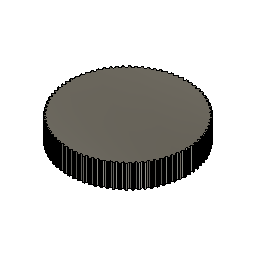
gear_82z (Autodesk Fusion 360 design; units mm, degrees)
Autodesk Fusion 360 part; units mm, degrees
sketch "Sketch1" plane through (0, 0, 0) normal (0, 0, 1) x (1, 0, 0) in component "gt2 pulley"
  circle A0 centre (0, 0) radius 26.1014 construction
  circle A1 centre (0, 0) radius 25.0974 construction
  line L0 (0, 0) -> (0, 26.1014) construction
  line L1 (0, 0) -> (0.9998, 26.0823) construction
  line L2 (0, 0) -> (1.4048, 26.0636) construction
  circle A2 centre (0, 0) radius 25.8474 construction
  arc A3 (0.396, 25.7111) -> (0.473, 25.4136) centre (1.3911, 25.8099) ccw
  circle A4 centre (0, 0) radius 25.6974 construction
  arc A5 (0.2481, 25.8462) -> (0, 25.8474) centre (0, 0) ccw
  arc A6 (0.396, 25.7111) -> (0.2481, 25.8462) centre (0.2468, 25.6962) ccw
  arc A7 (0.473, 25.4136) -> (0.9613, 25.079) centre (0.9826, 25.6336) ccw
  arc A8 (0, 25.8474) -> (-0.2481, 25.8462) centre (0, 0) ccw
  arc A9 (-0.2481, 25.8462) -> (-0.396, 25.7111) centre (-0.2468, 25.6962) ccw
  arc A10 (-0.473, 25.4136) -> (-0.396, 25.7111) centre (-1.3911, 25.8099) ccw
  arc A11 (-0.9613, 25.079) -> (-0.473, 25.4136) centre (-0.9826, 25.6336) ccw
  arc A12 (0.9613, 25.079) -> (-0.9613, 25.079) centre (0, 0) ccw
  point P0 (1.3911, 25.8099)
  point P1 (0, 25.8474)
  dimension "d18" = 52.2028
  dimension "d19" = 2.195
  dimension "d22" = 1.004
  dimension "d24" = 0.75
  dimension "d26" = 1
  dimension "d27" = 0.15
  dimension "d28" = 0.15
  dimension "d47" = 0.555
  dimension "d52" = 3.812
  constraint coincident A0.centre A1.centre
  constraint coincident A0 L0.end
  constraint vertical L0
  constraint coincident A0 L1.end
  constraint coincident A0 L2.end
  constraint concentric A1 A2
  constraint coincident A1 A7.end
  constraint coincident L1 A7.end
  constraint coincident A2 P0
  constraint coincident L2 P0
  constraint coincident P0 A3.centre
  constraint coincident A2 P1
  constraint coincident L0 P1
  constraint concentric A2 A4
  constraint coincident P1 A5.end
  constraint coincident A4 A6.centre
  constraint coincident A3.start A6.start
  constraint tangent A3 A6
  constraint tangent A3 A7
  constraint symmetric L0 A7.end A11.start
  constraint symmetric L0 A3.start A9.end
  constraint symmetric L0 A3.end A10.start
  constraint symmetric L0 A3 A10
  constraint symmetric L0 A5.start A8.end
  constraint symmetric L0 P1 A5.end
  constraint symmetric L0 A5 A8
  constraint symmetric L0 A6 A9
  constraint symmetric L0 A7 A11
  constraint coincident A1 A11.start
  constraint tangent A1 A7
  constraint coincident L1 A7.centre
  measures "d18" diameter of A0
  measures "d19" angle of L0 L1
  measures "d22" distance of A0 A1
  measures "d24" distance of A1 A2
  measures "d26" radius of A3
  measures "d27" distance of A2 A4
  measures "d28" radius of A6
  measures "d47" radius of A7
extrude "Extrude1" add sketch "Sketch1" along normal blind 10 makes body 1
pattern_circular "C-Pattern1" count 82 over 360 about axis through (0, 0, 1.75) along (0, 0, 1) of bodies 1 makes body 2 at (-2.0277, 25.0154, 6.6667) makes body 3 at (-3.9367, 24.7867, 6.6667) makes body 4 at (-5.8225, 24.4127, 6.6667) makes body 5 at (-8.2819, 23.6915, 6.6667) makes body 6 at (-8.6841, 23.5471, 3.3333) makes body 7 at (-11.6124, 22.2493, 6.6667) makes body 8 at (-12.1768, 21.9455, 3.3333) makes body 9 at (-13.821, 20.949, 6.6667) makes body 10 at (-16.0503, 19.2942, 6.6667) makes body 11 at (-16.8569, 18.5937, 3.3333) makes body 12 at (-18.8075, 16.618, 6.6667) makes body 13 at (-20.2791, 14.7864, 6.6667) makes body 14 at (-21.1238, 13.5523, 6.6667) makes body 15 at (-21.6814, 12.6411, 3.3333) makes body 16 at (-22.5854, 10.9443, 6.6667) makes body 17 at (-23.3569, 9.1833, 3.3333) makes body 18 at (-24.3877, 5.9264, 6.6667) makes body 19 at (-24.7698, 4.0421, 6.6667) makes body 20 at (-25.0065, 2.1342, 6.6667) makes body 21 at (-25.0965, 0.2137, 6.6667) makes body 22 at (-25.0965, -0.2137, 3.3333) makes body 23 at (-25.0065, -2.1342, 3.3333) makes body 24 at (-24.485, -5.5103, 6.6667) makes body 25 at (-23.9914, -7.3684, 6.6667) makes body 26 at (-23.4343, -8.9841, 6.6667) makes body 27 at (-22.5854, -10.9443, 6.6667) makes body 28 at (-21.6814, -12.6411, 6.6667) makes body 29 at (-21.463, -13.0084, 3.3333) makes body 30 at (-19.6315, -15.636, 6.6667) makes body 31 at (-18.2307, -17.2488, 6.6667) makes body 32 at (-17.9344, -17.5567, 3.3333) makes body 33 at (-16.5378, -18.878, 6.6667) makes body 34 at (-14.8726, -20.216, 6.6667) makes body 35 at (-12.3632, -21.841, 6.6667) makes body 36 at (-10.655, -22.7234, 6.6667) makes body 37 at (-8.6841, -23.5471, 6.6667) makes body 38 at (-6.8561, -24.1428, 6.6667) makes body 39 at (-6.4441, -24.256, 3.3333) makes body 40 at (-4.5684, -24.6781, 3.3333) makes body 41 at (-1.1748, -25.0699, 6.6667) makes body 42 at (-0.1068, -25.0972, 6.6667) makes body 43 at (1.1748, -25.0699, 3.3333) makes body 44 at (3.9367, -24.7867, 6.6667) makes body 45 at (5.8225, -24.4127, 6.6667) makes body 46 at (8.2819, -23.6915, 6.6667) makes body 47 at (8.6841, -23.5471, 3.3333) makes body 48 at (11.6124, -22.2493, 6.6667) makes body 49 at (12.917, -21.5182, 6.6667) makes body 50 at (13.821, -20.949, 6.6667) makes body 51 at (16.0503, -19.2942, 6.6667) makes body 52 at (16.8569, -18.5937, 3.3333) makes body 53 at (19.2257, -16.1323, 6.6667) makes body 54 at (20.2791, -14.7864, 6.6667) makes body 55 at (21.463, -13.0084, 6.6667) makes body 56 at (22.0992, -11.8956, 6.6667) makes body 57 at (22.8576, -10.364, 6.6667) makes body 58 at (23.3569, -9.1833, 3.3333) makes body 59 at (24.2284, -6.5473, 6.6667) makes body 60 at (24.7698, -4.0421, 6.6667) makes body 61 at (24.835, -3.6198, 3.3333) makes body 62 at (25.0392, -1.7081, 3.3333) makes body 63 at (25.0965, 0.2137, 3.3333) makes body 64 at (24.9193, 2.9844, 6.6667) makes body 65 at (24.485, 5.5103, 6.6667) makes body 66 at (23.9914, 7.3684, 6.6667) makes body 67 at (23.8624, 7.7758, 3.3333) makes body 68 at (23.1972, 9.5797, 6.6667) makes body 69 at (22.3958, 11.3273, 3.3333) makes body 70 at (21.0076, 13.7317, 6.6667) makes body 71 at (19.8948, 15.2995, 6.6667) makes body 72 at (18.2307, 17.2488, 6.6667) makes body 73 at (17.9344, 17.5567, 3.3333) makes body 74 at (16.5378, 18.878, 6.6667) makes body 75 at (14.5263, 20.4663, 6.6667) makes body 76 at (12.3632, 21.841, 6.6667) makes body 77 at (10.655, 22.7234, 6.6667) makes body 78 at (9.2827, 23.3176, 6.6667) makes body 79 at (6.8561, 24.1428, 6.6667) makes body 80 at (5.6145, 24.4614, 6.6667) makes body 81 at (3.0904, 24.9064, 6.6667) makes body 82 at (1.1748, 25.0699, 6.6667)
sketch "Sketch2" plane through (0, 0, 10) normal (0, 0, 1) x (-1, 0, 0)
  arc A0 (-11.7634, -22.8656) -> (-11.6908, -23.0524) centre (-11.6231, -22.9186) ccw
  arc A1 (-11.6908, -23.0524) -> (-11.2461, -23.2726) centre (0, 0) ccw
  arc A2 (-11.2461, -23.2726) -> (-11.0536, -23.2171) centre (-11.1808, -23.1376) ccw
  arc A3 (-10.8526, -22.9847) -> (-11.0536, -23.2171) centre (-10.2057, -23.7473) ccw
  arc A4 (-10.2666, -22.9015) -> (-10.8526, -22.9847) centre (-10.4936, -23.4079) ccw
  arc A5 (-11.9895, -22.0484) -> (-10.2666, -22.9015) centre (0, 0) ccw
  arc A6 (-11.7004, -22.5649) -> (-11.9895, -22.0484) centre (-12.2547, -22.536) ccw
  arc A7 (-11.7634, -22.8656) -> (-11.7004, -22.5649) centre (-12.6991, -22.5127) ccw
  circle A8 centre (0, 0) radius 25.0974
  constraint concentric A1 A8
extrude "Extrude2" add sketch "Sketch2" against normal blind 10 contours A5 A8 bodies 1 2 3 4 5 6 7 8 9 10 11 12 13 14 15 16 17 18 19 20 21 22 23 24 25 26 27 28 29 30 31 32 33 34 35 36 37 38 39 40 41 42 43 44 45 46 47 48 49 50 51 52 53 54 55 56 57 58 59 60 61 62 63 64 65 66 67 68 69 70 71 72 73 74 75 76 77 78 79 80 81 82
extrude "Extrude4" [suppressed] in component "gt2 pulley"
pattern_circular "C-Pattern7" [suppressed] in component "gt2 pulley"
extrude "Extrude3" [suppressed] in component "gt2 pulley"
pattern_circular "C-Pattern6" [suppressed] in component "gt2 pulley"
extrude "Extrude2'" [suppressed] in component "gt2 pulley"
pattern_circular "C-Pattern5" [suppressed] in component "gt2 pulley"
extrude "Extrude1'" [suppressed] in component "gt2 pulley"
pattern_circular "C-Pattern4" [suppressed] in component "gt2 pulley"
pattern_circular "C-Pattern3" [suppressed] in component "gt2 pulley"
pattern_circular "C-Pattern2" [suppressed] in component "gt2 pulley"
pattern_circular "C-Pattern1'" [suppressed] in component "gt2 pulley"
copy_body "Body->Comp1" [suppressed] in component "Component"
copy_body "Body->Comp2" [suppressed] in component "Component'"
copy_body "Body->Comp3" [suppressed] in component "Component''"
copy_body "Body->Comp4" [suppressed] in component "Component'''"
copy_body "Body->Comp5" [suppressed] in component "Component''''"
copy_body "Body->Comp6" [suppressed] in component "Component'''''"
copy_body "Body->Comp7" [suppressed] in component "Component''''''"
copy_body "Body->Comp8" [suppressed] in component "Component'''''''"
copy_body "Body->Comp9" [suppressed] in component "Component''''''''"
copy_body "Body->Comp10" [suppressed] in component "Component'''''''''"
copy_body "Body->Comp11" [suppressed] in component "Component''''''''''"
copy_body "Body->Comp12" [suppressed] in component "Component'''''''''''"
copy_body "Body->Comp13" [suppressed] in component "Component''''''''''''"
copy_body "Body->Comp14" [suppressed] in component "Component'''''''''''''"
copy_body "Body->Comp15" [suppressed] in component "Component''''''''''''''"
copy_body "Body->Comp16" [suppressed] in component "Component'''''''''''''''"
copy_body "Body->Comp17" [suppressed] in component "Component''''''''''''''''"
copy_body "Body->Comp18" [suppressed] in component "Component'''''''''''''''''"
copy_body "Body->Comp19" [suppressed] in component "Component''''''''''''''''''"
copy_body "Body->Comp20" [suppressed] in component "Component'''''''''''''''''''"
component "gt2 pulley" placed x (1, 0, 0) y (0, 1, 0) z (0, 0, 1) at (0, 0, 0)
equation "NumTeeth = 82" comment "min 20"
equation "ToothPitch = 2 mm"
equation "PullyDia = NumTeeth * ToothPitch / PI"
equation "ToothAng = ( ( 360 / NumTeeth ) * 1 deg )"
equation "TransOffsetAngle = ToothAng * 0.2"
equation "Sholulder_Radius = 0.15 mm"
equation "Root_Radius = 0.555 mm"
equation "TransRadius = 1 mm"
equation "ToolHeight = 0.75 mm"
equation "PLD = 0.254 mm"
equation "d18 = PullyDia"
equation "d19 = ToothAng / 2"
equation "d22 = PLD + ToolHeight"
equation "d24 = ToolHeight"
equation "d26 = TransRadius"
equation "d27 = Sholulder_Radius"
equation "d31 = NumTeeth"
equation "d33 = NumTeeth"
equation "d35 = NumTeeth"
equation "d37 = NumTeeth"
equation "d41 = NumTeeth"
equation "d45 = NumTeeth"
equation "d47 = Root_Radius"
equation "d50 = NumTeeth"
